Autodesk Inventor part; units mm, degrees
(part 2 of 2)
  arc A621 (20.3804, 2.2111) -> (20.3335, 2.6078) centre (0, 0) ccw
  arc A622 (20.1441, 3.8033) -> (20.0662, 4.1951) centre (0, 0) ccw
  arc A623 (19.7836, 5.372) -> (19.6752, 5.7565) centre (0, 0) ccw
  arc A624 (19.3011, 6.9077) -> (19.1629, 7.2825) centre (0, 0) ccw
  arc A625 (18.6997, 8.4007) -> (18.5324, 8.7635) centre (0, 0) ccw
  arc A626 (17.9829, 9.842) -> (17.7877, 10.1905) centre (0, 0) ccw
  arc A627 (17.1553, 11.2226) -> (16.9334, 11.5547) centre (0, 0) ccw
  arc A628 (16.2219, 12.534) -> (15.9746, 12.8477) centre (0, 0) ccw
  arc A629 (15.1885, 13.7681) -> (14.9173, 14.0614) centre (0, 0) ccw
  arc A630 (14.0614, 14.9173) -> (13.7681, 15.1885) centre (0, 0) ccw
  arc A631 (12.8477, 15.9746) -> (12.534, 16.2219) centre (0, 0) ccw
  arc A632 (11.5547, 16.9334) -> (11.2226, 17.1553) centre (0, 0) ccw
  arc A633 (10.1905, 17.7877) -> (9.842, 17.9829) centre (0, 0) ccw
  arc A634 (8.7635, 18.5324) -> (8.4007, 18.6997) centre (0, 0) ccw
  arc A635 (7.2825, 19.1629) -> (6.9077, 19.3011) centre (0, 0) ccw
  arc A636 (5.7565, 19.6752) -> (5.372, 19.7836) centre (0, 0) ccw
  arc A637 (4.1951, 20.0662) -> (3.8033, 20.1441) centre (0, 0) ccw
  arc A638 (2.6078, 20.3335) -> (2.2111, 20.3804) centre (0, 0) ccw
  arc A639 (1.0044, 20.4754) -> (0.6052, 20.4911) centre (0, 0) ccw
  point P0 (0, 0)
  constraints: 960 point on circle, 480 centre point, 2 horizontal alignment, 2 vertical alignment, 476 other
extrude "Extrusion1" add sketch "Sketch1" against normal blind 3
body "Solid1"
